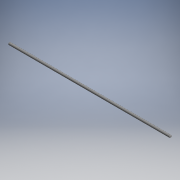
# Autodesk Inventor part: PSFG6-400
Saved by Autodesk Inventor 2017.3 (Build 213256000, 256)
## iProperties
Part Number: PSFG6-400
Material: Generic
Catalog Web Link: www.cadenas.de
Description: SFJ, SFU, SSFJ, SSFU, PSFJ, PSFU, PSSFJ, PSSFU, RSFJ, RSSFJ, PSFG, PSSFG-Shafts - Solid Type
Vendor: MISUMI
Document SubType Name: Modeling
Designer: partserver
Manufacturer: MISUMI
Mass: 11.3053 g
Surface Area: 75.8468 cm^2
Volume: 11.3053 cm^3
Density: 1 g/cm^3
Appearance: PSOLRGB-175-175-175
Category: PARTsolutions
Company: MISUMI
Title: PSFG6-400
Author: Cadenas PARTsolutions
Comments: Shafts - Solid Type
PSOL_IDENT_0: {$CADENAS_DATA\23d-libs\misumi\metric\01_linear_shafts\sfj.prj},373 {VTYP=3D},{NB=PSFG6-400},{LINA=P
PSOL_IDENT_1: SFG6-400},{NN=SFJ, SFU, SSFJ, SSFU, PSFJ, PSFU, PSSFJ, PSSFU, RSFJ, RSSFJ, PSFG, PSSFG},{DATE=31.08.
PSOL_IDENT_2: 2021 14:41:00},{GEOMDATE=25.08.2021 09:43:46},{VERSION=},{LINEID=40},{WBVAR=DTS,MAT,ST,ALT1,L,ALT3,S
PSOL_IDENT_3: C,WSC,X,ALT4,FC,WFC,A,E,ALT5,RC,WRC,Y,ALT6,VC,WVC,F,ALT7,KC,G,WKC,CALT7},{WBNUMERIC=L,SC,WSC,X,FC,WF
PSOL_IDENT_4: C,A,E,RC,WRC,Y,VC,WVC,F,KC,G,WKC,CALT7}  {NB=PSFG6-400},{LINA=PSFG6-400},{KT=DUMMY},{PN=PSFG6-400},{
PSOL_IDENT_5: TYPE=PSFG},{DTS=f8},{DTSALG= 'g6','g6' , 'h5','h5' , 'f8','f8' },{MAT=S45C},{MATALG= 'S45C','S45C Eq
PSOL_IDENT_6: uivalent','SUS304','304 Stainless Steel' },{ST=HCP10},{STALG= 'HCP10','Hard Chrome Plating Plating H
PSOL_IDENT_7: ardness: HV750 ~ Plating Thickness: 10 microns or More' },{D=6},{ALT1=},{ALT1ALG= '','w/o LKC (L Dim
PSOL_IDENT_8: ension Tolerance Change)','LKC','with LKC (L Dimension Tolerance Change)' },{ALT1PN=},{L=400.0},{LAL
PSOL_IDENT_9: G=[15:900/1]},{LMIN=15},{LMAX=900},{C=0.5},{ALT3=},{ALT3ALG= '','w/o Wrench Flats' , 'SC','with SC (
PSOL_IDENT_10: Wrench Flats at One Location)' , 'WSC','with WSC (Wrench Flats at Two Locations)' },{ALT3PN=},{SC=0}
PSOL_IDENT_11: ,{SCALG=[0]},{SCMAX=392},{WSC=0},{WSCALG=[0]},{WSCMAX=382},{X=0},{XALG=[0]},{XMAX=382},{WALT3=0},{LL
PSOL_IDENT_12: 1=0},{LL1ALG=8},{ALT4=},{ALT4ALG= '','w/o Set Screw Flat','FC','with FC (Set Screw Flat at One Locat
PSOL_IDENT_13: ion)','WFC','with WFC (Set Screw Flats at Two Locations)' },{ALT4PN=},{FC=0},{FCALG=[0]},{FCMAX=30},
PSOL_IDENT_14: {WFC=0},{WFCALG=[0]},{WFCMAX=30},{A=0},{AALG=[0]},{AMAX=0},{E=0},{EALG=[0]},{EMAX=398},{HHALT4=0.0},
PSOL_IDENT_15: {CIFA=0},{CIFE=0},{FC3D=0},{ALT5=},{ALT5ALG= '','Not applicable' },{ALT5PN=},{RC=0},{RCALG=[0]},{RCM
PSOL_IDENT_16: IN=2},{RCMAX=400},{WRC=0},{WRCALG=[0]},{WRCMIN=2},{WRCMAX=396},{Y=0},{YALG=[0]},{YMIN=2},{YMAX=398},
PSOL_IDENT_17: {BB1=0},{BB1ALG=0},{HHALT5=0.0},{ALT6=},{ALT6ALG= '','w/o V Groove','VC','with VC (V Groove at One L
PSOL_IDENT_18: ocation)','WVC','with WVC (V Grooves at Two Locations)' },{ALT6PN=},{VC=0},{VCALG=[0]},{VCMIN=3},{VC
PSOL_IDENT_19: MAX=398},{WVC=0},{WVCALG=[0]},{WVCMIN=2},{WVCMAX=395},{F=0},{FALG=[0]},{FMIN=3},{FMAX=398},{WALT6=0}
PSOL_IDENT_20: ,{WALT6ALG=2},{ALT7=},{ALT7ALG= '','Not applicable' },{ALT7PN=},{KC=0},{KCALG=[0]},{KCMAX1=398},{KCM
PSOL_IDENT_21: AX2=400},{KCMAX3=398},{G=0},{GALG=[0]},{GMIN=0},{GMAX1=30},{GMAX2=30},{GMAX3=30},{WKC=0},{WKCALG=[0]
PSOL_IDENT_22: },{WKCMAX=398},{CALT7=0},{CALT7ALG=[0]},{CALT7MIN=0},{CALT7MAX=30},{BB=0},{TT=0.0},{CIFKC=0},{CIFWKC=
PSOL_IDENT_23: 0},{ERRORPN=},{ERRORALT34=OK},{ERRORALT35=OK},{ERRORALT36=OK},{ERRORALT37=OK},{ERRORALT45=OK},{ERROR
PSOL_IDENT_24: ALT46=OK},{ERRORALT47=OK},{ERRORALT56=OK},{ERRORALT57=OK},{ERRORALT67=OK},{FONTSIZE=0.720}
NB: PSFG6-400
NN: SFJ, SFU, SSFJ, SSFU, PSFJ, PSFU, PSSFJ, PSSFU, RSFJ, RSSFJ, PSFG, PSSFG
NT: Shafts - Solid Type
NBSYN: $PN.
LINA: PSFG6-400
CATALOG: Misumi
PN: PSFG6-400
DTS: f8
MAT: S45C Equivalent
ST: Hard Chrome Plating Plating Hardness: HV750 ~ Plating Thickness: 10 microns or More
D: 6
ALT1: w/o LKC (L Dimension Tolerance Change)
L: 400
C: 0.5
ALT3: w/o Wrench Flats
SC: 0
WSC: 0
X: 0
WALT3: 0
LL1: 0
ALT4: w/o Set Screw Flat
FC: 0
WFC: 0
A: 0
E: 0
HHALT4: 0
ALT5: Not applicable
RC: 0
WRC: 0
Y: 0
BB1: 0
HHALT5: 0
ALT6: w/o V Groove
VC: 0
WVC: 0
F: 0
WALT6: 0
ALT7: Not applicable
KC: 0
G: 0
WKC: 0
CALT7: 0
BB: 0
TT: 0
SUPPLIER: MISUMI
ARTICLENO: PSFG6-400
BOMINFO: PSFG6-400
CREATOR: CADENAS GmbH
Autodesk Inventor part; units mm, degrees
ref_plane "YZ Plane" through (0, 0, 0) normal (1, 0, 0) x (0, 1, 0)
ref_plane "XZ Plane" through (0, 0, 0) normal (0, 1, 0) x (-1, 0, 0)
ref_plane "XY Plane" through (0, 0, 0) normal (0, 0, 1) x (1, 0, 0)
sketch "Sketch_3" plane through (0, 0, 0) normal (0, 0, 1) x (1, 0, 0)
  line L0 (400, 0) -> (0, 0)
  line L1 (0, 0) -> (0, 2.5)
  line L2 (0, 2.5) -> (0.5, 3)
  line L3 (0.5, 3) -> (399.5, 3)
  line L4 (399.5, 3) -> (400, 2.5)
  line L5 (400, 2.5) -> (400, 0)
  line L6 (400, 0) -> (0, 0)
  constraints: 14 end point
revolve "Revolution1" add sketch "Sketch_3" angle 360 about axis through (400, 0, 0) along (1, 0, 0)
body "Solid1"
